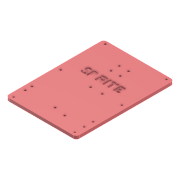
# Autodesk Inventor part: top plate
Saved by Autodesk Inventor 2022 (Build 260153000, 153)
## iProperties
Created: 2024-03-20
Part Number: top plate
Material: Generic
Document SubType Name: Modeling
Designer: david
Density: 1 g/cm^3
Appearance: Smooth - Red
Author: david
Autodesk Inventor part; units mm, degrees
ref_plane "YZ Plane" through (0, 0, 0) normal (1, 0, 0) x (0, 1, 0)
ref_plane "XZ Plane" through (0, 0, 0) normal (0, 1, 0) x (-1, 0, 0)
ref_plane "XY Plane" through (0, 0, 0) normal (0, 0, 1) x (1, 0, 0)
sketch "Sketch1" plane through (0, 0, 0) normal (0, 1, 0) x (-1, 0, 0)
  line L0 (57.5, -160) -> (57.5, -160) construction
  line L1 (-57.5, -160) -> (-57.5, 0) construction
  line L2 (-57.5, 0) -> (57.5, 0)
  line L3 (57.5, 0) -> (57.5, -160) construction
  line L4 (80.5, 0) -> (-80.5, 0) construction
  line L5 (0, -192) -> (0, 32) construction
  line L6 (57.5, -160) -> (-57.5, -160)
  line L7 (-57.5, -160) -> (-57.5, -160) construction
  line L8 (57.5, 0) -> (-55.1767, 0)
  line L9 (57.5, -40) -> (-57.5, -40) construction
  line L10 (-57.5, -40) -> (-57.5, 0)
  line L11 (-57.5, 0) -> (57.5, 0)
  line L12 (57.5, 0) -> (57.5, -40)
  line L13 (-57.5, -160) -> (-57.5, -40)
  line L14 (57.5, -160) -> (57.5, -40)
  point P0 (0, 0)
  dimension "width" = 115
  dimension "Length" = 160
  dimension "d2" = 115
  dimension "d112" = 40
  constraints: 26 end point, 6 parallel, 5 horizontal, 4 perpendicular, 1 collinear, 1 point on line, 1 symmetric about line, 1 vertical alignment, 1 other
  measures "width" distance of L1.end L2.end
  measures "Length" distance of L1.start L1.end
  measures "d2" distance of L6.end L0.end
  measures "d112" distance between parallel lines of L2 L9
extrude "Base" add sketch "Sketch1" against normal blind 5
sketch "Sketch11" plane through (0, 0, 0) normal (0, 1, 0) x (1, 0, 0)
  line L0 (0, 218.4) -> (0, -36.4) construction
  line L1 (-57.5, 0) -> (57.5, 0) construction
  line L2 (57.5, 160) -> (-57.5, 160) projected
  line L3 (-50, 5) -> (50, 5) construction
  line L4 (50, 5) -> (50, 35) construction
  line L5 (50, 35) -> (-50, 35) construction
  line L6 (-50, 35) -> (-50, 5) construction
  point P0 (0, 0)
  point P1 (50, 155)
  point P2 (-50, 155)
  dimension "d91" = 5
  dimension "d92" = 50
  dimension "d93" = 5
  dimension "d94" = 50
  dimension "d113" = 30
  constraints: 8 end point, 2 coincident, 2 parallel, 2 symmetric about line, 1 horizontal, 1 perpendicular, 1 vertical alignment
  measures "d91" distance from line of L1 point (50, 5)
  measures "d92" distance from line of point (50, 5) L0
  measures "d93" distance from line of L2 point (50, 155)
  measures "d94" distance from line of L0 point (50, 155)
  measures "d113" distance of L3.end L4.end
hole "Mounting Holes" at (50, 0, -5) at (-50, 0, -5) at (50, 0, -155) at (-50, 0, -155) at (-50, 0, -35) at (50, 0, -35) direction (0, -1, 0) diameter 3.4 depth 6
fillet "Fillet1" radius 5 4 edges at (-57.5, -2.5, 0) (57.5, -2.5, -160) (-57.5, -2.5, -160) (57.5, -2.5, 0)
sketch "Sketch12" plane through (0, 0, 0) normal (0, 1, 0) x (1, 0, 0)
  line L0 (-50, 82) -> (-1, 82) construction
  line L1 (-1, 82) -> (-1, 24) construction
  line L2 (-1, 24) -> (-50, 24) construction
  line L3 (-50, 24) -> (-50, 82) construction
  line L4 (-57.5, 155) -> (-57.5, 5) projected
  line L5 (0, 218.4) -> (0, -36.4) projected
  line L6 (-52.5, 0) -> (52.5, 0) projected
  circle A0 centre (-50, 35) radius 1.7 projected
  point P0 (0, 0)
  point P1 (0, 0)
  point P2 (52.2987, 0)
  point P3 (-57.5, 40)
  point P4 (0, 0)
  dimension "d103" = 49
  dimension "d104" = 58
  dimension "d239" = 24
  constraints: 8 end point, 2 parallel, 1 horizontal, 1 midpoint, 1 perpendicular, 1 vertical alignment
  measures "d103" distance of L1.end L2.end
  measures "d104" distance of L0.end L1.end
  measures "d239" distance between parallel lines of L6 L2
hole "RasPi Mounting Holes" at (-50, 0, -82) at (-1, 0, -82) at (-1, 0, -24) at (-50, 0, -24) direction (0, -1, 0) diameter 3.4 depth 6
sketch "Sketch15" plane through (0, 0, 0) normal (0, 1, 0) x (1, 0, 0)
  line L0 (50, 82) -> (50, 20.5) construction
  line L1 (50, 20.5) -> (18, 20.5) construction
  line L2 (18, 20.5) -> (18, 82) construction
  line L3 (18, 82) -> (50, 82) construction
  line L4 (-52.5, 0) -> (52.5, 0) projected
  circle A0 centre (-1, 82) radius 1.7 projected
  circle A1 centre (50, 35) radius 1.7 projected
  point P0 (0, 0)
  point P1 (0, 0)
  dimension "d122" = 32
  dimension "d123" = 61.5
  constraints: 8 end point, 4 coincident, 2 parallel, 1 horizontal alignment, 1 midpoint, 1 perpendicular, 1 vertical, 1 vertical alignment
  measures "d122" distance of L2.end L0.start
  measures "d123" distance of L1.end L2.end
hole "LM2596 Mounting Holes" at (50, 0, -82) at (50, 0, -20.5) at (18, 0, -20.5) at (18, 0, -82) direction (0, -1, 0) diameter 3.4 depth 6
sketch "Sketch16" plane through (0, 0, 0) normal (0, 1, 0) x (1, 0, 0)
  line L0 (-7.5, 122) -> (7.5, 122) construction
  line L1 (7.5, 122) -> (7.5, 135.5) construction
  line L2 (7.5, 135.5) -> (-7.5, 135.5) construction
  line L3 (-7.5, 135.5) -> (-7.5, 122) construction
  line L4 (52.5, 160) -> (-52.5, 160) projected
  point P0 (0, 0)
  point P1 (0, 135.5)
  point P2 (0, 160)
  dimension "d132" = 15
  dimension "d133" = 13.5
  dimension "d251" = 24.5
  constraints: 8 end point, 4 coincident, 2 midpoint, 2 parallel, 1 horizontal, 1 perpendicular, 1 vertical alignment
  measures "d132" distance of L1.end L2.end
  measures "d133" distance of L2.end L0.start
  measures "d251" distance between parallel lines of L2 L4
hole "Camera Mount Mounting Holes" at (-7.5, 0, -135.5) at (-7.5, 0, -122) at (7.5, 0, -122) at (7.5, 0, -135.5) direction (0, -1, 0) diameter 3.4 depth 6
sketch "Sketch17" plane through (0, 0, 0) normal (0, 1, 0) x (1, 0, 0)
  line L0 (-57.1973, 19.3379) -> (-57.1973, 79.4802) construction
  line L1 (-57.1973, 79.4802) -> (-14.6793, 79.4802) construction
  line L2 (-14.6793, 79.4802) -> (-14.6793, 19.3379) construction
  line L3 (-14.6793, 19.3379) -> (-57.1973, 19.3379) construction
  circle A0 centre (-50, 24) radius 1.7 projected
  circle A1 centre (-50, 82) radius 1.7 projected
  line L4 (-52.5, 0) -> (52.5, 0) projected
  spline S0 degree 4 poles (-23.5768, 107.5562) (-23.9599, 108.1329) (-26.7206, 109.5318) (-29.2007, 109.4276) (-31.1711, 108.3992) (-32.4678, 106.727) (-32.6924, 104.8622) (-31.7857, 101.8118) (-28.8011, 101.2833) (-23.9996, 100.1938) (-27.1532, 96.7821) (-29.6649, 98.5187) (-31.4067, 99.7767) knots 0 0 0 0 0 0.20272 0.281354 0.355201 0.433005 0.51958 0.610323 0.697239 0.780233 1 1 1 1 1
  line L5 (-31.4067, 99.7767) -> (-32.9921, 97.7539)
  line L6 (-23.5768, 107.5562) -> (-24.9607, 105.3771)
  spline S1 degree 4 poles (-24.9607, 105.3771) (-25.575, 105.6423) (-26.0812, 106.4667) (-28.8483, 107.206) (-30.1427, 105.6184) (-29.5307, 104.2217) (-27.3268, 103.8879) (-26.61, 103.5516) (-24.6737, 102.912) (-23.5813, 101.615) (-23.0114, 100.5309) (-23.3364, 97.2492) (-26.4089, 95.0894) (-31.046, 95.5958) (-32.5754, 97.531) (-32.9921, 97.7539) knots 0 0 0 0 0 0.144957 0.205265 0.266901 0.324627 0.385746 0.449034 0.509011 0.57578 0.647336 0.728379 0.816759 1 1 1 1 1
  line L7 (-22.3201, 108.9601) -> (-22.3201, 95.9175)
  line L8 (-22.3201, 95.9175) -> (-19.5912, 95.9248)
  line L9 (-19.5912, 95.9248) -> (-19.5912, 99.7767)
  line L10 (-19.5815, 106.4203) -> (-19.5815, 102.3589)
  line L11 (-19.5815, 102.3589) -> (-17.2644, 102.3589)
  line L12 (-19.5815, 106.4203) -> (-17.2644, 106.4203)
  line L13 (-22.3201, 108.9601) -> (-17.1865, 108.9601)
  line L14 (-19.5912, 99.7767) -> (-17.1865, 99.7767)
  spline S2 degree 4 poles (-17.1865, 108.9601) (-15.7222, 109.1611) (-13.0222, 108.3576) (-12.2123, 103.6083) (-13.2625, 101.3351) (-15.0817, 99.7415) (-17.1865, 99.7767) knots 0 0 0 0 0 0.423309 0.583119 1 1 1 1 1
  spline S3 degree 4 poles (-17.2644, 106.4203) (-15.8013, 106.6282) (-14.2337, 104.6304) (-15.4318, 102.4479) (-17.2644, 102.3589) knots 0 0 0 0 0 1 1 1 1 1
  line L15 (-8.892, 105.1807) -> (-8.892, 95.9035)
  line L16 (-8.892, 95.9035) -> (-5.5761, 95.9035)
  line L17 (-5.5761, 95.9035) -> (-5.5761, 96.079)
  line L18 (-5.5761, 96.079) -> (-5.5761, 99.8252)
  line L19 (-5.5761, 99.8252) -> (-3.8649, 99.8252)
  line L20 (-3.8649, 99.8252) -> (-1.345, 95.9035)
  line L21 (-1.345, 95.9035) -> (2.6566, 95.9035)
  line L22 (2.6566, 95.9035) -> (0.1367, 99.8252)
  line L23 (-8.892, 105.1807) -> (-5.5761, 105.1807)
  line L24 (-5.5761, 105.1807) -> (-5.5761, 103.2106)
  line L25 (-5.5761, 103.2106) -> (-1.6405, 103.2106)
  line L26 (-1.6405, 103.2106) -> (-1.6405, 105.7998)
  line L27 (-1.6405, 105.7998) -> (-8.892, 105.7998)
  line L28 (-8.892, 105.7998) -> (-8.892, 109.1077)
  line L29 (-8.892, 109.1077) -> (0.4248, 109.1077)
  line L30 (1.7311, 107.6584) -> (1.7311, 101.4882)
  arc A2 (0.1367, 99.8252) -> (1.7311, 101.4882) centre (0, 101.5521) ccw
  arc A3 (1.7311, 107.6584) -> (0.4248, 109.1077) centre (-0.6091, 106.8624) ccw
  line L31 (3.6229, 109.1077) -> (6.9877, 109.1077)
  line L32 (6.9877, 109.1077) -> (6.9877, 95.9035)
  line L33 (6.9877, 95.9035) -> (3.6229, 95.9035)
  line L34 (3.6229, 95.9035) -> (3.6229, 109.1077)
  line L35 (8.5216, 109.1077) -> (8.5216, 105.7998)
  line L36 (8.5216, 105.7998) -> (11.8904, 105.7998)
  line L37 (11.8904, 105.7998) -> (11.8904, 95.9035)
  line L38 (11.8904, 95.9035) -> (15.2013, 95.9035)
  line L39 (15.2013, 95.9035) -> (15.2013, 109.1077)
  line L40 (15.2013, 109.1077) -> (8.5216, 109.1077)
  line L41 (15.8152, 109.1077) -> (15.8152, 105.7998)
  line L42 (15.8152, 105.7998) -> (18.2596, 105.7998)
  line L43 (18.2596, 105.7998) -> (20.5061, 109.1077)
  line L44 (20.5061, 109.1077) -> (15.8152, 109.1077)
  line L45 (21.1807, 109.1139) -> (21.1807, 95.9035)
  line L46 (21.1807, 95.9035) -> (24.5026, 95.9035)
  line L47 (24.5026, 95.9035) -> (24.5026, 109.1139)
  line L48 (24.5026, 109.1139) -> (21.1807, 109.1139)
  line L49 (25.078, 104.1957) -> (25.078, 100.8438)
  line L50 (25.078, 100.8438) -> (27.5701, 100.8438)
  line L51 (27.5701, 100.8438) -> (27.5701, 104.1957)
  line L52 (27.5701, 104.1957) -> (25.078, 104.1957)
  line L53 (24.5026, 109.1139) -> (24.5026, 105.7759)
  line L54 (24.5026, 105.7759) -> (29.6113, 105.7759)
  line L55 (29.6113, 105.7759) -> (29.6113, 109.1139)
  line L56 (29.6113, 109.1139) -> (24.5026, 109.1139)
  line L57 (29.6113, 109.1139) -> (31.7796, 105.7759)
  line L58 (31.7796, 105.7759) -> (29.6113, 105.7759)
  line L59 (27.5701, 104.1957) -> (29.7825, 104.1679)
  line L60 (29.7825, 104.1679) -> (27.5701, 100.8438)
  line L61 (24.5026, 99.2428) -> (31.7797, 99.2428)
  line L62 (31.7797, 99.2428) -> (29.6113, 95.9035)
  line L63 (29.6113, 95.9035) -> (24.5026, 95.9035)
  line L64 (-19.5912, 95.9248) -> (-6.4294, 95.9248)
  line L65 (-57.5, 155) -> (-57.5, 5) projected
  line L66 (57.5, 5) -> (57.5, 155) projected
  line L67 (57.5, 155) -> (57.5, 5) projected
  point P0 (0, 0)
  point P1 (-35.9383, 19.3379)
  point P2 (0, 0)
  point P3 (-25.1122, 108.5587)
  point P4 (-27.9572, 109.2621)
  point P5 (-31.105, 108.2479)
  point P6 (-32.4933, 105.0039)
  point P7 (-28.329, 101.1439)
  point P8 (-25.978, 99.9423)
  point P9 (-26.2061, 98.7647)
  point P10 (-27.977, 98.1297)
  point P11 (-31.4836, 102.4672)
  point P12 (-32.1758, 106.8515)
  point P13 (-29.8122, 108.9936)
  point P14 (-25.7492, 105.8825)
  point P15 (-27.2147, 106.5554)
  point P16 (-29.1272, 106.4629)
  point P17 (-29.8182, 105.5604)
  point P18 (-29.3344, 104.5209)
  point P19 (-27.5574, 103.8728)
  point P20 (-26.4604, 103.5224)
  point P21 (-24.8384, 102.7794)
  point P22 (-23.7279, 101.7052)
  point P23 (-23.248, 100.5646)
  point P24 (-23.568, 97.9839)
  point P25 (-25.7498, 96.0066)
  point P26 (-29.7351, 95.9082)
  point P27 (-32.2992, 97.2048)
  point P28 (-14.7056, 108.4809)
  point P29 (-13.0519, 106.5426)
  point P30 (-12.7004, 104.0446)
  point P31 (-13.1129, 102.2581)
  point P32 (-14.2816, 100.7542)
  point P33 (-15.9909, 105.993)
  point P34 (-15.3145, 104.6743)
  point P35 (-15.7107, 103.1836)
  constraints: 120 end point, 8 point on line, 4 point on circle, 2 centre point, 2 midpoint, 2 vertical, 1 horizontal, 50 other
extrude "SP RITE" cut sketch "Sketch17" against normal blind 2 contours L6 S1 L5 S0 | L13 S2 L14 L9 L8 L7 | L12 S3 L11 L10 | L23 L24 L25 L26 L27 L28 L29 A3 L30 A2 L22 L21 L20 L19 L18 L17 L16 L15 | L31 L32 L33 L34 | L40 L39 L38 L37 L36 L35 | L44 L43 L42 L41 | L48 L47 L46 L45 | L56 L55 L54 L47 | L47 L61 L62 L63 | L57 L58 L55 | L52 L51 L50 L49 | L59 L60 L51
equation "\"d2\" = width"
equation "\"d94\" = d92"
equation "\"d95\" = HoleDia"
equation "\"d105\" = HoleDia"
equation "\"d125\" = HoleDia"
equation "\"d135\" = HoleDia"
equation "\"HoleDia\" = 3.4"
body "Solid1"
